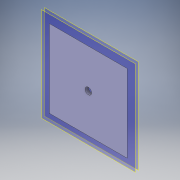
# Autodesk Inventor part: insulationlid
Saved by Autodesk Inventor 2018 (Build 220112000, 112)
## iProperties
Created: 2019-02-19
Part Number: insulationlid
Material: Generic
Document SubType Name: Modeling
Designer: F8PLTW
Density: 1 g/cm^3
Appearance: Default
Author: F8PLTW
Autodesk Inventor part; units mm, degrees
ref_plane "YZ Plane" through (0, 0, 0) normal (1, 0, 0) x (0, 1, 0)
ref_plane "XZ Plane" through (0, 0, 0) normal (0, 1, 0) x (-1, 0, 0)
ref_plane "XY Plane" through (0, 0, 0) normal (0, 0, 1) x (1, 0, 0)
sketch "Sketch1" plane through (0, 0, 0) normal (0, 0, 1) x (1, 0, 0)
  line L0 (-11.214, 10.6272) -> (138.786, 10.6272)
  line L1 (138.786, 10.6272) -> (138.786, -139.3728)
  line L2 (138.786, -139.3728) -> (-11.214, -139.3728)
  line L3 (-11.214, -139.3728) -> (-11.214, 10.6272)
  point P0 (0, 0)
  dimension "d0" = 150
  dimension "d1" = 150
  constraints: 8 end point, 2 parallel, 1 horizontal, 1 perpendicular
  measures "d0" distance of L1.end L2.end
  measures "d1" distance of L0.end L1.end
ref_plane "Work Plane2" through (-11.214, 10.6272, -6.35) normal (0, 0, -1) x (1, 0, 0)
ref_plane "Work Plane1" through (-11.214, 10.6272, 0) normal (0, 0, -1) x (1, 0, 0)
sketch "Sketch2" plane through (-11.214, 10.6272, -6.35) normal (0, 0, -1) x (1, 0, 0)
  line L0 (143.6624, 6.35) -> (6.3624, 6.35)
  line L1 (6.3624, 6.35) -> (6.3624, 143.65)
  line L2 (6.3624, 143.65) -> (143.6624, 143.65)
  line L3 (143.6624, 143.65) -> (143.6624, 6.35)
  line L4 (150, 0) -> (0, 0) construction
  line L5 (0, 0) -> (0, 150) construction
  point P0 (11.214, 10.6272)
  dimension "d3" = 137.3
  dimension "d4" = 137.3
  dimension "d6" = 6.35
  dimension "d7" = 143.6624
  constraints: 12 end point, 3 horizontal, 2 parallel, 2 perpendicular, 1 vertical
  measures "d3" distance of L1.end L2.end
  measures "d4" distance of L0.end L1.end
  measures "d6" distance between parallel lines of L4 L0
  measures "d7" distance between parallel lines of L5 L3
loft "Loft1" add profiles "Sketch1", "Sketch2"
sketch "Sketch3" plane through (-11.214, 10.6272, 0) normal (0, 0, 1) x (1, 0, 0)
  line L0 (0, 0) -> (6.3624, -6.35) projected
  line L1 (150, 0) -> (150, -150) projected
  line L2 (0, 0) -> (150, -150) construction
  line L3 (0, -150) -> (6.3624, -143.65) projected
  line L4 (0, -150) -> (150, 0) construction
  circle A0 centre (75, -75) radius 6.35
  point P0 (11.214, -10.6272)
  dimension "d12" = 12.7
  constraints: 4 end point, 1 centre point, 1 midpoint
  measures "d12" diameter of A0
extrude "Extrusion1" cut sketch "Sketch3" against normal blind 25.4
body "Solid1"
